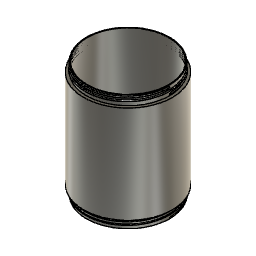
Container (Autodesk Fusion 360 design; units mm, degrees)
Autodesk Fusion 360 part; units mm, degrees
sketch "Sketch1" plane through (0, 0, 0) normal (0, 0, 1) x (1, 0, 0)
  circle A0 centre (0, 0) radius 57.5
  circle A1 centre (0, 0) radius 55
  circle A2 centre (0, 0) radius 53.75
  circle A3 centre (0, 0) radius 52.75
  dimension "d4" = 110
  dimension "d57" = 115
  dimension "d60" = 107.5
  dimension "d63" = 105.5
  constraint coincident A0.centre A1.centre
  constraint concentric A0 A2
  constraint concentric A0 A3
  measures "d4" diameter of A1
  measures "d57" diameter of A0
  measures "d60" diameter of A2
  measures "d63" diameter of A3
extrude "Extrude8" add sketch "Sketch1" along normal blind 150 contours A2
ref_plane "WorkPlane6" through (0, 0, 140) normal (0, 0, 1) x (1, 0, 0)
coil "CoilPrimitive5" add diameter 107.5 section circle size 2 on centre turns 2 pitch 4 right hand placed x (1, 0, 0) y (0, 1, 0) z (0, 0, 1) at (0, 0, 140)
fillet "Fillet8" radius 0.95 4 edges at (54.4571, 0, 148.7071) (54.4571, 0, 147.2929) (54.4571, 0, 140.7071) (54.4571, 0, 139.2929)
ref_plane "WorkPlane7" through (0, 0, 1) normal (0, 0, 1) x (1, 0, 0)
coil "CoilPrimitive6" add diameter 107.5 section circle size 1.5 on centre turns 2 pitch 4 right hand placed x (1, 0, 0) y (0, 1, 0) z (0, 0, 1) at (0, 0, 1)
fillet "Fillet9" radius 0.7 2 edges at (54.2803, 0, 1.5303) (54.2803, 0, 0.4697)
fillet "Fillet10" radius 0.7 2 edges at (54.2803, 0, 9.5303) (54.2803, 0, 8.4697)
ref_plane "WorkPlane8" through (0, 0, 12) normal (0, 0, 1) x (1, 0, 0)
sketch "Sketch9" plane through (0, 0, 12) normal (0, 0, 1) x (1, 0, 0)
  circle A0 centre (0, 0) radius 57.5
  circle A1 centre (0, 0) radius 53.75
  dimension "d89" = 115
  dimension "d90" = 107.5
  constraint coincident A0.centre A1.centre
  constraint concentric A0 A1
  measures "d89" diameter of A0
  measures "d90" diameter of A1
extrude "Extrude11" add sketch "Sketch9" along normal blind 126
ref_plane "WorkPlane9" through (0, 0, 15) normal (0, 0, 1) x (1, 0, 0)
sketch "Sketch13" plane through (0, 0, 15) normal (0, 0, 1) x (1, 0, 0)
ref_plane "WorkPlane10" through (0, 0, 25) normal (0, 0, 1) x (1, 0, 0)
sketch "Sketch14" plane through (0, 0, 25) normal (0, 0, 1) x (1, 0, 0)
  circle A0 centre (0, 0) radius 55
  dimension "d95" = 110
  constraint coincident A0.centre origin
  measures "d95" diameter of A0
equation "d4 = 115 mm - 5 mm"
equation "d63 = 107.5 mm - 2 mm"
equation "d68 = 150 mm - 10 mm"
equation "d91 = 150 mm - 12 mm - 12 mm"
equation "d83 = ( 5.8 / 2 ) * 1 mm"
equation "d89 = ( 21 / 2 ) * 1 mm"
equation "d33 = 90 deg + 13.9 deg"
equation "d35 = 71.259 mm + 6 mm"
